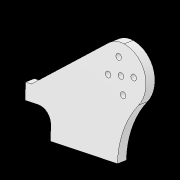
# Autodesk Inventor part: UHMWMotorUpright
Saved by Autodesk Inventor 2022 (Build 260153000, 153)
## iProperties
Created: 2021-02-15
Part Number: UHMWMotorUpright
Material: UHMW, White
Document SubType Name: Modeling
Designer: Esketitttttt
Density: 0.94 g/cm^3
Appearance: Smooth - White
Mass: 16.3377 g
Surface Area: 73.6215 cm^2
Volume: 17.3805 cm^3
heightForAxle: 1.748 in
Author: Esketitttttt
Autodesk Inventor part; units mm, degrees
ref_plane "YZ Plane" through (0, 0, 0) normal (1, 0, 0) x (0, 1, 0)
ref_plane "XZ Plane" through (0, 0, 0) normal (0, 1, 0) x (-1, 0, 0)
ref_plane "XY Plane" through (0, 0, 0) normal (0, 0, 1) x (1, 0, 0)
sketch "Sketch1" plane through (0, 0, 0) normal (1, 0, 0) x (0, 1, 0)
  circle A0 centre (-42.9876, 10.1686) radius 1.25
  circle A1 centre (-35.154, 0.6082) radius 1.25
  circle A2 centre (-45.7852, -5.696) radius 1.25
  circle A3 centre (-53.6188, 3.8643) radius 1.25
  line L0 (0.0001, -0.0006) -> (0.0001, 61.1604)
  line L1 (0.0001, 2.2363) -> (-44.3864, 2.2363) construction
  circle A4 centre (-44.3864, 2.2363) radius 1.7145
  line L2 (-35.154, 0.6082) -> (-44.3864, 2.2363) construction
  line L3 (-44.3864, 2.2363) -> (-42.9876, 10.1686) construction
  line L4 (-42.9876, 10.1686) -> (-44.3864, 2.2363) construction
  line L5 (-53.6188, 3.8643) -> (-44.3864, 2.2363) construction
  line L6 (-45.7852, -5.696) -> (-44.3864, 2.2363) construction
  line L7 (-0.0009, 51.5412) -> (-7.9999, 51.5413) construction
  arc A5 (-9.9999, 53.5413) -> (-7.9999, 51.5413) centre (-7.9999, 53.5413) ccw construction
  line L8 (-9.9999, 53.5413) -> (-9.9999, 61.1604) construction
  line L9 (-9.9999, 61.1604) -> (-31.7499, 61.1604)
  line L10 (-31.7499, 61.1604) -> (-31.7499, 61.1604)
  line L11 (-65.1399, 0.3814) -> (0.0001, 0.3814) construction
  circle A6 centre (-8.1189, 53.0414) radius 8.119
  line L12 (0.0001, 61.1604) -> (-9.9999, 61.1604)
  line L13 (-8.1189, 53.0414) -> (-8.1189, 61.1604)
  line L14 (-8.1189, 61.1604) -> (0.0001, 61.1604)
  line L15 (-8.1189, 44.9224) -> (0.0001, 44.9224)
  line L16 (-16.2379, 53.0414) -> (-16.2379, 61.1604)
  line L17 (0.0001, 61.1604) -> (0.0001, 3.1704)
  circle A7 centre (-44.3864, 2.2363) radius 17.0996 construction
  line L18 (0.0001, 3.1704) -> (-37.4698, -13.402) construction
  circle A8 centre (-44.3864, 2.2363) radius 49.4644 construction
  line L19 (-31.7499, 61.1604) -> (-31.7499, 57.4908)
  line L20 (-31.7499, 57.4908) -> (-25.3999, 57.4908)
  line L21 (-25.3999, 57.4908) -> (-25.3999, 61.1604)
  line L22 (-25.3999, 61.1604) -> (-31.7499, 61.1604)
  line L23 (-31.7499, 61.1604) -> (-31.7499, 57.4908)
  line L24 (-25.3999, 57.4908) -> (-58.6623, 10.6274)
  circle A9 centre (-44.3864, 2.2363) radius 15.6 construction
  line L25 (-44.3864, 2.2363) -> (-27.5466, -0.7333) construction
  line L26 (-44.3864, 2.2363) -> (-61.2261, 5.2059) construction
  line L27 (-44.3864, 2.2363) -> (-47.356, -14.6035) construction
  arc A10 (-47.0956, -13.1267) -> (-27.5466, -0.7333) centre (-44.1134, 3.784) ccw
  arc A11 (-61.2261, 5.2059) -> (-47.0956, -13.1267) centre (-44.1134, 3.784) ccw
  line L28 (-44.3864, 2.2363) -> (-41.6772, 17.5992) construction
  arc A12 (-41.6772, 17.5992) -> (-61.2261, 5.2059) centre (-44.6593, 0.6885) ccw
  arc A13 (-27.5466, -0.7333) -> (-41.6772, 17.5992) centre (-44.6593, 0.6885) ccw
  line L29 (0.0001, 3.1704) -> (-25.3999, 3.1704) construction
  arc A14 (0.0001, 3.1704) -> (-32.8146, -9.1466) centre (0.0001, -46.7004) ccw
  point P0 (0, 0)
  point P1 (-14.2875, 38.1)
  point P2 (0.0001, 51.16)
  point P3 (0.0002, 21.2479)
  point P4 (0.0001, 44.9224)
  point P5 (-27.3877, 0.3814)
  point P6 (-6.3058, 0.3814)
  point P7 (0.0001, 53.0414)
  dimension "d0" = 44.3865
  dimension "d1" = 3.429
  dimension "d2" = 9.3749
  dimension "d3" = 8.0547
  dimension "d4" = 9.3749
  dimension "d5" = 8.0547
  dimension "d6" = 16.238
  dimension "d7" = 8.119
  dimension "d8" = 57.99
  dimension "d9" = 34.1992
  dimension "d29" = 98.9288
  dimension "d30" = 31.75
  dimension "d42" = 44.3865
  dimension "d43" = 3.6695
  dimension "d44" = 58.9241
  dimension "d45" = 6.35
  dimension "d46" = 31.2
  dimension "d47" = 100.001
  dimension "d48" = 100.001
  dimension "d49" = 25.4
  dimension "d65" = 2.5
  constraints: 60 end point, 27 point on circle, 15 centre point, 10 point on line, 10 tangent, 8 perpendicular, 7 horizontal, 5 coincident, 4 vertical, 3 equal radius, 2 parallel, 1 collinear
  measures "d0" distance of L1.start L1.end
  measures "d1" diameter of A4
  measures "d2" distance of L2.start L5.end
  measures "d3" distance of L5.end L3.end
  measures "d4" distance of L5.start L5.end
  measures "d5" distance of L6.start L5.end
  measures "d6" diameter of A6
  measures "d7" distance of L0.end L13.end
  measures "d8" distance of L0.end L17.end
  measures "d9" diameter of A7
  measures "d29" diameter of A8
  measures "d30" distance between parallel lines of L10 L17
  measures "d42" horizontal distance of L0.end L1.end
  measures "d43" distance of L10.end L19.end
  measures "d44" distance of L0.end L1.start
  measures "d45" distance of L22.end L21.end
  measures "d46" diameter of A9
  measures "d47" angle of L27 L1
  measures "d48" angle of L1 L6
  measures "d49" distance of L17.end L29.end
  measures "d65" diameter of A2
extrude "Extrusion1" add sketch "Sketch1" along normal blind 6.35 contours A14 A10 A13 A12 L24 L21 L9 L16 A6 L15 L0 | A10 A11 A12 A13
sketch "Sketch2" plane through (6.35, 0, 0) normal (1, 0, 0) x (0, 0, -1)
  line L0 (-14.3281, -60.9849) -> (-12.7, -51.7525)
  line L1 (-56.5983, -32.7278) -> (-22.8866, -67.8945)
  arc A0 (-22.8866, -67.8945) -> (-21.3075, -68.315) centre (-21.3075, -65.14) ccw
  circle A1 centre (-14.3281, -60.9849) radius 1.25
  line L2 (-12.7, -51.7525) -> (-20.6323, -50.3537)
  line L3 (-20.6323, -50.3537) -> (-12.7, -51.7525)
  line L4 (-4.7677, -53.1513) -> (-12.7, -51.7525)
  arc A2 (-3.175, -68.315) -> (0, -65.14) centre (-3.175, -65.14) ccw
  line L5 (-21.3075, -68.315) -> (-3.175, -68.315)
  circle A3 centre (-12.7, -51.7525) radius 3.175
  circle A4 centre (-4.7677, -53.1513) radius 1.25
  circle A5 centre (-20.6323, -50.3537) radius 1.25
  circle A6 centre (-11.0719, -42.5201) radius 1.25
  line L6 (0, -65.14) -> (0, 0)
  line L7 (-12.7, 0) -> (-12.7, -51.7525) construction
  line L8 (-11.0719, -42.5201) -> (-12.7, -51.7525)
  line L9 (0, 0) -> (-61.16, 0)
  line L10 (0, 0) -> (-51.16, 0)
  arc A7 (-56.5983, -32.7278) -> (-58.8903, -31.75) centre (-58.8903, -34.925) ccw
  line L11 (-61.16, -31.75) -> (-58.8903, -31.75)
  arc A8 (-53.16, -10) -> (-51.16, -8) centre (-53.16, -8) ccw construction
  line L12 (-61.16, -10) -> (-61.16, -31.75)
  line L13 (-53.16, -10) -> (-61.16, -10) construction
  line L14 (-51.16, 0) -> (-51.16, -8) construction
  circle A9 centre (-52.66, -12.7) radius 8.5
  line L15 (-61.16, 0) -> (-61.16, -10)
  line L16 (-52.66, -12.7) -> (-61.16, -12.7)
  line L17 (-61.16, -12.7) -> (-61.16, 0)
  line L18 (-44.16, -12.7) -> (-44.16, 0)
  line L19 (-52.66, -21.2) -> (-61.16, -21.2)
  line L20 (-61.16, 0) -> (-21.2475, 0)
  circle A10 centre (-12.7, -51.7525) radius 19.6052
  line L21 (-21.2475, 0) -> (4.0472, -41.5596)
  line L22 (-61.1604, -16.2379) -> (-61.1604, -25.3999) projected
  point P0 (-38.1, -14.2875)
  point P1 (-51.16, 0)
  point P2 (-21.2475, 0)
  point P3 (-44.16, 0)
  point P4 (-30.5153, -59.9366)
  point P5 (-61.16, -31.75)
  point P6 (-61.1604, -31.7499)
  dimension "d21" = 39.2104
  dimension "d12" = 51.7525
  dimension "d13" = 6.35
  dimension "d14" = 9.3749
  dimension "d15" = 8.0547
  dimension "d16" = 9.3749
  dimension "d17" = 8.0547
  dimension "d18" = 17
  dimension "d19" = 12.7
  dimension "d20" = 39.9125
  constraints: 44 end point, 11 point on circle, 10 centre point, 6 perpendicular, 4 point on line, 2 coincident, 2 tangent, 1 collinear, 5 other
  measures "d12" distance of L7.start L7.end
  measures "d13" diameter of A3
  measures "d14" distance of L8.start L0.end
  measures "d15" distance of L0.end L2.end
  measures "d16" distance of L0.start L0.end
  measures "d17" distance of L4.start L0.end
  measures "d18" diameter of A9
  measures "d19" distance of L16.end L17.end
  measures "d20" distance of L17.end L20.end
hole "Hole1" [suppressed]
sketch "Sketch4" plane through (6.35, 0, 0) normal (1, 0, 0) x (0, 0, -1)
  line L0 (-3.1704, 0.0001) -> (-44.9224, 0.0001) projected
  line L1 (-44.9224, 0.0001) -> (-44.9224, -8.1189) projected
  arc A0 (-53.0414, -16.2379) -> (-44.9224, -8.1189) centre (-53.0414, -8.1189) ccw projected
  line L2 (-53.0414, -16.2379) -> (-61.1604, -16.2379) projected
  line L3 (-61.1604, -25.3999) -> (-57.4908, -25.3999) projected
  line L4 (-35.4535, -9.5249) -> (-26.3909, -9.5249)
  arc A1 (-26.3909, -9.5249) -> (-14.3756, -46.6234) centre (46.0656, -6.553) ccw
  arc A2 (-13.4746, -47.6813) -> (-14.3756, -46.6234) centre (-10.5479, -44.2762) ccw
  arc A3 (-15.8585, -54.8082) -> (-13.4746, -47.6813) centre (-16.8369, -50.5188) ccw
  line L5 (-15.8585, -54.8082) -> (-45.5241, -24.0814)
  arc A4 (-45.5241, -24.0814) -> (-35.4535, -9.5249) centre (-53.0414, -8.1189) ccw
  circle A5 centre (-20.6323, -50.3537) radius 2.7135 projected
  line L6 (-22.2573, -48.1806) -> (-28.8731, -41.3281)
  line L7 (-28.8731, -41.3281) -> (-21.1207, -33.8435) construction
  arc A6 (-28.8731, -41.3281) -> (-21.1207, -33.8435) centre (-26.5003, -36.0286) ccw
  line L8 (-61.1604, -16.2379) -> (-61.1604, -25.3999) projected
  arc A7 (-5.2059, -61.2261) -> (9.1466, -32.8146) centre (-3.784, -44.1134) ccw projected
  arc A8 (-3.1704, 0.0001) -> (9.1466, -32.8146) centre (46.7004, 0.0001) ccw projected
  line L9 (-57.4908, -25.3999) -> (-10.6274, -58.6623) projected
  arc A9 (-10.6274, -58.6623) -> (-5.2059, -61.2261) centre (-0.6885, -44.6593) ccw projected
  point P0 (0, 0)
  dimension "d51" = 9.525
  dimension "d52" = 9.525
  constraints: 11 point on circle, 8 end point, 5 centre point, 2 point on line, 1 perpendicular, 1 tangent, 2 other
  measures "d51" distance between parallel lines of L0 L4
  measures "d52" distance of L6.start L6.end
extrude "Pocketing" [suppressed]
fillet "Fillet1" [suppressed]
sketch "Sketch3" plane through (0, 0.0001, 44.9224) normal (0, 1, 0) x (1, 0, 0)
  line L0 (0, 0) -> (6.35, 0)
  line L1 (3.175, 0) -> (3.175, 13.9173) construction
  line L2 (3.175, 13.9173) -> (3.175, 27.8347) construction
  line L3 (0, 41.752) -> (6.35, 41.752) projected
  line L4 (0, 41.752) -> (0, 0) projected
  point P0 (0, 8.119)
  dimension "d33" = 13.9173
  dimension "d34" = 13.9173
  dimension "d50" = 41.752
  dimension "d56" = 3.175
  constraints: 6 end point, 2 coincident, 2 vertical, 1 horizontal, 1 midpoint
  measures "d33" distance of L1.start L1.end
  measures "d34" distance of L1.end L2.end
  measures "d50" distance between parallel lines of L3 L0
  measures "d56" distance between parallel lines of L4 L1
hole "Hole2" at (3.175, 0.0001, 31.005) at (3.175, 0.0001, 17.0877) direction (0, -1, 0) diameter 2.9464 depth 9.525 tip angle 118
sketch "Sketch5" plane through (6.35, 0, 0) normal (1, 0, 0) x (0, 0, -1)
  circle A0 centre (-0.6082, -35.154) radius 1.25 projected
  circle A1 centre (-10.1686, -42.9876) radius 1.25 projected
  circle A2 centre (5.696, -45.7852) radius 1.25 projected
  circle A3 centre (-3.8643, -53.6188) radius 1.25 projected
  point P0 (0, 0)
hole "Hole3" at (6.35, -35.154, 0.6082) at (6.35, -45.7852, -5.696) at (6.35, -42.9876, 10.1686) at (6.35, -53.6188, 3.8643) direction (-1, 0, 0) diameter 3.5 end through all countersink diameter 5.427 countersink angle 90
sketch "Sketch6" plane through (0, 0, 0) normal (-1, 0, 0) x (0, 0, 1)
  line L0 (61.1604, -25.3999) -> (57.4908, -25.3999) projected
  line L1 (53.0414, -16.2379) -> (61.1604, -16.2379) projected
  arc A0 (44.9224, -8.1189) -> (53.0414, -16.2379) centre (53.0414, -8.1189) ccw projected
  line L2 (44.9224, 0.0001) -> (44.9224, -8.1189) projected
  line L3 (3.1704, 0.0001) -> (44.9224, 0.0001) projected
  line L4 (61.1604, -16.2379) -> (61.1604, -25.3999) projected
  arc A1 (-9.1466, -32.8146) -> (5.2059, -61.2261) centre (3.784, -44.1134) ccw projected
  arc A2 (5.2059, -61.2261) -> (10.6274, -58.6623) centre (0.6885, -44.6593) ccw projected
  line L5 (57.4908, -25.3999) -> (10.6274, -58.6623) projected
  arc A3 (-9.1466, -32.8146) -> (3.1704, 0.0001) centre (-46.7004, 0.0001) ccw projected
  point P0 (0, 0)
fillet "Fillet2" radius 12.7 1 edges at (3.175, -61.2261, 5.2059)
equation "\"d7\" = 0.5 * d6"
equation "\"heightForAxle\" = 44.3865"
body "Solid1"
